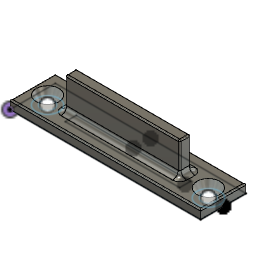
barn-door-lower-slot-floor-guide-v3 (Autodesk Fusion 360 design; units mm, degrees)
Autodesk Fusion 360 part; units mm, degrees
sketch "Sketch1" plane through (0, 0, 0) normal (0, 1, 0) x (1, 0, 0)
  line L0 (0, 0) -> (83.4, 0)
  line L1 (83.4, 0) -> (83.4, 19.8)
  line L2 (83.4, 19.8) -> (0, 19.8)
  line L3 (0, 19.8) -> (0, 0)
  circle A0 centre (6.5, 9.9) radius 5
  circle A1 centre (76.9, 9.9) radius 5
  line L4 (16.7, 12.3) -> (66.7, 12.3)
  line L5 (66.7, 12.3) -> (66.7, 7.5)
  line L6 (66.7, 7.5) -> (16.7, 7.5)
  line L7 (16.7, 7.5) -> (16.7, 12.3)
  circle A2 centre (76.9, 9.9) radius 2.8
  circle A3 centre (6.5, 9.9) radius 2.8
  point P0 (66.7, 9.9)
  point P1 (83.4, 9.9)
  point P2 (41.7, 12.3)
  point P3 (41.7, 19.8)
  dimension "d1" = 83.4
  dimension "d2" = 19.8
  dimension "d3" = 10
  dimension "d4" = 6.5
  dimension "d5" = 10
  dimension "d6" = 6.5
  dimension "d7" = 50
  dimension "d9" = 4.8
  dimension "d18" = 5.6
  dimension "d19" = 5.6
  constraint horizontal L0
  constraint vertical L1
  constraint horizontal L2
  constraint vertical L3
  constraint coincident L0.start L3.end
  constraint horizontal L4
  constraint vertical L5
  constraint horizontal L6
  constraint vertical L7
  constraint midpoint L5 P0
  constraint midpoint L1 P1
  constraint horizontal P0 P1
  constraint midpoint L4 P2
  constraint midpoint L2 P3
  constraint vertical P2 P3
  constraint concentric A1 A2
  constraint concentric A0 A3
  measures "d1" distance of L1.end L2.end
  measures "d2" distance of L0.end L1.end
  measures "d3" diameter of A0
  measures "d4" distance of L3 A0.centre
  measures "d5" diameter of A1
  measures "d6" distance of L1 A1.centre
  measures "d7" distance of L4.start L4.end
  measures "d9" distance of L4.start L6.end
  measures "d18" diameter of A2
  measures "d19" diameter of A3
extrude "Extrude1" add sketch "Sketch1" along normal blind 17.8 contours L4 L5 L6 L7 makes body 1
extrude "Extrude2" add sketch "Sketch1" along normal blind 3.8 separate body contours L0 L1 L2 L3 makes body 2
extrude "Extrude3" add sketch "Sketch1" along normal blind 3.8 separate body contours A0 | A1 | A2 | A3 makes body 3 at (81.8938, 1.2667, -9.6508) makes body 4 at (11.4752, 2.5333, -9.4022)
extrude "Extrude4" cut sketch "Sketch1" along normal blind 3.8 draft 30 contours A2 | A3 bodies 3 4
combine "Combine1" operation add target body 2 tool bodies 1
combine "Combine2" operation add target body 2 tool bodies 3 4
fillet "Fillet1" radius 0.6 12 edges at (66.7, 10.8, -12.3) (66.7, 10.8, -7.5) (41.7, 17.8, -12.3) (83.4, 3.8, -9.9) (41.7, 3.8, -19.8) (41.7, 3.8, 0) (66.7, 17.8, -9.9) (16.7, 17.8, -9.9) (0, 3.8, -9.9) (41.7, 17.8, -7.5) (16.7, 10.8, -7.5) (16.7, 10.8, -12.3) on bodies 2
fillet "Fillet2" radius 2.5 8 edges at (66.5243, 3.8, -12.1243) (66.7, 3.8, -9.9) (66.5243, 3.8, -7.6757) (41.7, 3.8, -7.5) (16.8757, 3.8, -7.6757) (16.7, 3.8, -9.9) (16.8757, 3.8, -12.1243) (41.7, 3.8, -12.3) on bodies 2
equation "d3 = screw_top_opening_width"
equation "d5 = screw_top_opening_width"
equation "plate_height = 3.8 mm"
equation "d14 = 14 mm + plate_height"
equation "d16 = plate_height"
equation "d18 = screw_bottom_opening_width"
equation "d19 = screw_bottom_opening_width"
equation "screw_top_opening_width = 10 mm"
equation "screw_bottom_opening_width = 5.6 mm"
equation "d22 = plate_height"
equation "d24 = plate_height"
equation "screw_taper_angle = 30 deg"
equation "outside_fillet_radiu = 0.6 mm"
equation "d29 = outside_fillet_radiu"
equation "inside_fillet_radius = 2.5 mm"
equation "d32 = inside_fillet_radius"
